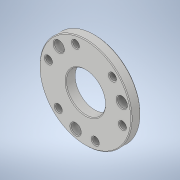
# Autodesk Inventor part: Motor_Adapter_Flex
Saved by Autodesk Inventor 2021 (Build 250183000, 183)
## iProperties
Created: 2020-10-12
Part Number: Motor_Adapter_Flex
Material: Generic
Document SubType Name: Modeling
Designer: PhotonUser
Density: 1 g/cm^3
Appearance: Default
Author: PhotonUser
Autodesk Inventor part; units mm, degrees
ref_plane "YZ Plane" through (0, 0, 0) normal (1, 0, 0) x (0, 1, 0)
ref_plane "XZ Plane" through (0, 0, 0) normal (0, 1, 0) x (-1, 0, 0)
ref_plane "XY Plane" through (0, 0, 0) normal (0, 0, 1) x (1, 0, 0)
sketch "Sketch1" plane through (0, 0, 0) normal (1, 0, 0) x (0, 1, 0)
  line L0 (0, 0) -> (47.0027, 0)
  line L1 (47.0027, 0) -> (47.0027, -9.525)
  line L2 (47.0027, -9.525) -> (0, -9.525)
  line L3 (0, -9.525) -> (0, 0)
  dimension "d0" = 47.0027
  dimension "d1" = 9.525
  constraints: 8 end point, 3 perpendicular, 1 horizontal
  measures "d0" distance of L0.start L0.end
  measures "d1" distance of L0.end L1.end
revolve "Revolution1" add sketch "Sketch1" angle 360 about axis through (0, 0, -9.525) along (0, 0, 1)
sketch "Sketch2" plane through (0, 0, 0) normal (0, 0, 1) x (1, 0, 0)
  circle A0 centre (0, 0) radius 39.0906
  line L0 (0, 0) -> (27.6412, 27.6412)
  line L1 (0, 0) -> (39.0906, 0) construction
  circle A1 centre (27.6412, 27.6412) radius 3.4036
  circle A2 centre (37.7586, -10.1174) radius 3.4036
  circle A3 centre (10.1174, -37.7586) radius 3.4036
  circle A4 centre (-27.6412, -27.6412) radius 3.4036
  circle A5 centre (-37.7586, 10.1174) radius 3.4036
  circle A6 centre (-10.1174, 37.7586) radius 3.4036
  point P0 (0, 0)
  dimension "d3" = 78.1812
  dimension "d4" = 45
  dimension "d5" = 6.8072
  dimension "d8" = 360
  constraints: 6 centre point, 4 end point, 2 coincident, 1 equal length, 1 horizontal, 16 other
  measures "d4" angle of L1 L0
  measures "d5" diameter of A1
extrude "Extrusion1" cut sketch "Sketch2" against normal blind 9.525 contours A1 L0 A0 | A0 A1 | A2 A0 | A0 A2 | L0 A1 A0 | A3 A0 | A0 A3 | A6 A0 | A0 A6 | A4 A0 | A0 A4 | A5 A0 | A0 A5
sketch "Sketch3" plane through (0, 0, 0) normal (0, 0, 1) x (1, 0, 0)
  circle A0 centre (0, 0) radius 38.481
  line L0 (0, 0) -> (-27.2102, 27.2102)
  line L1 (0, 0) -> (38.481, 0) construction
  circle A1 centre (-27.6412, -27.6412) radius 3.4036 projected
  circle A2 centre (-27.2102, 27.2102) radius 5.08
  circle A3 centre (-9.9596, -37.1698) radius 5.08
  circle A4 centre (37.1698, 9.9596) radius 5.08
  circle A5 centre (0, 0) radius 19.939
  point P0 (0, 0)
  dimension "d12" = 76.962
  dimension "d13" = 135
  dimension "d14" = 10.16
  dimension "d17" = 360
  dimension "d21" = 39.878
  constraints: 4 centre point, 4 end point, 3 coincident, 1 equal length, 1 horizontal, 10 other
  measures "d13" angle of L1 L0
  measures "d14" diameter of A2
  measures "d21" diameter of A5
extrude "Extrusion2" cut sketch "Sketch3" against normal blind 9.525 contours A4 A0 | A0 A4 | A3 A0 | A0 A3 | A2 L0 A0 | A0 A2 | L0 A2 A0 | A5
chamfer "Chamfer1" distance 0.762 angle 45 12 edges at (-19.939, 0, 0) (0, -47.0027, 0) (0, -47.0027, -9.525) (32.0898, 9.9596, 0) (24.2376, 27.6412, 0) (-13.521, 37.7586, 0) (-32.2902, 27.2102, 0) (-41.1622, 10.1174, 0) (-31.0448, -27.6412, 0) (-15.0396, -37.1698, 0) (6.7138, -37.7586, 0) (34.355, -10.1174, 0)
body "Solid1"
